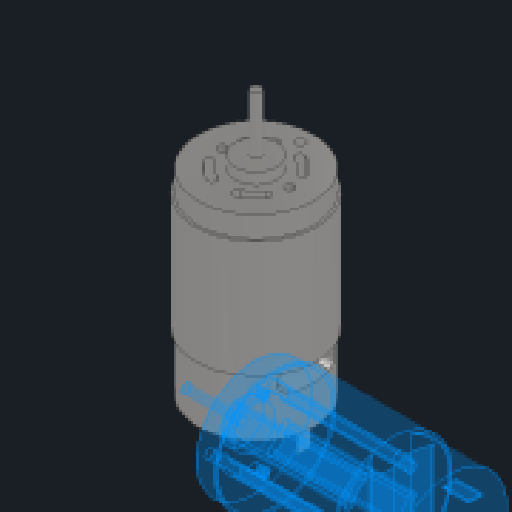
# Autodesk Inventor part: rs390
Saved by Autodesk Inventor 2023 (Build 270158000, 158)
## iProperties
Created: 2024-04-13
Part Number: rs390
Material: Steel, Mild
Document SubType Name: Modeling
Designer: szymo
Density: 3.82207 g/cm^3
Appearance: Semi-Polished
Mass: 100 g
Surface Area: 88.1627 cm^2
Volume: 26.1638 cm^3
Author: szymo
Autodesk Inventor part; units mm, degrees
ref_plane "YZ Plane" through (0, 0, 0) normal (1, 0, 0) x (0, 1, 0)
sketch "Sketch1" plane through (0, 0, 0) normal (0, 1, 0) x (-1, 0, 0)
  circle A0 centre (0, 0) radius 13.7
  dimension "d0" = 27.4
  constraints: 1 centre point, 1 coincident
  measures "d0" diameter of A0
extrude "Extrusion1" add sketch "Sketch1" along normal blind 46.5
sketch "Sketch2" plane through (0, 46.5, 0) normal (0, 1, 0) x (1, 0, 0)
  circle A0 centre (0, 0) radius 13.7 projected
  circle A1 centre (0, 0) radius 5
  dimension "d3" = 10
  constraints: 1 centre point, 1 coincident
  measures "d3" diameter of A1
extrude "Extrusion2" add sketch "Sketch2" along normal blind 2.7 contours A1
sketch "Sketch3" plane through (0, 46.5, 0) normal (0, 1, 0) x (1, 0, 0)
  circle A0 centre (0, 0) radius 5 projected
  circle A1 centre (0, 0) radius 5 projected
  circle A2 centre (0, 0) radius 13.7 projected
  circle A3 centre (0, 0) radius 13.7 projected
  line L0 (-13.7, 0) -> (13.7, 0)
  point P0 (-8, 0)
  point P1 (8, 0)
  dimension "d6" = 16
  dimension "d7" = 5.7
  dimension "d8" = 5.7
  constraints: 2 end point, 2 point on circle, 2 point on line, 1 horizontal
  measures "d6" distance of point (-8, 0) point (8, 0)
  measures "d7" distance of L0.start point (-8, 0)
  measures "d8" distance of L0.end point (8, 0)
hole "Hole1" at (-8, 46.5, 0) at (8, 46.5, 0) direction (0, -1, 0) diameter 2.1129 depth 2.8 thread size "M2.6x0.45" class "6H" standard "ISO Metric profile"
ref_plane "Work Plane1" through (0, 41.5, 0) normal (0, 1, 0) x (1, 0, 0)
sketch "Sketch4" plane through (0, 41.5, 0) normal (0, 1, 0) x (1, 0, 0)
  circle A0 centre (0, 0) radius 14.375
  dimension "d17" = 28.75
  constraints: 1 centre point, 1 coincident
  measures "d17" diameter of A0
extrude "Extrusion3" add sketch "Sketch4" against normal blind 27.7
sketch "Sketch5" plane through (0, 0, 0) normal (0, -1, 0) x (1, 0, 0)
  circle A0 centre (0, 0) radius 5
  dimension "d20" = 10
  constraints: 1 centre point, 1 coincident
  measures "d20" diameter of A0
extrude "Extrusion4" add sketch "Sketch5" along normal blind 4
sketch "Sketch6" plane through (0, 0, 0) normal (0, -1, 0) x (1, 0, 0)
  circle A0 centre (0, 0) radius 5 projected
  circle A1 centre (0, 0) radius 5 projected
  circle A2 centre (0, 0) radius 13.7 projected
  circle A3 centre (0, 0) radius 13.7 projected
  line L0 (13.7, 0) -> (-13.7, 0)
  line L1 (-11.5, 1.5) -> (-12, 1.5)
  line L2 (-12, 1.5) -> (-12, -1.5)
  line L3 (-12, -1.5) -> (-11.5, -1.5)
  line L4 (-11.5, -1.5) -> (-11.5, 1.5)
  line L5 (11.5, 1.5) -> (11, 1.5)
  line L6 (11, 1.5) -> (11, -1.5)
  line L7 (11, -1.5) -> (11.5, -1.5)
  line L8 (11.5, -1.5) -> (11.5, 1.5)
  dimension "d23" = 22.5
  dimension "d24" = 0.5
  dimension "d25" = 0.5
  dimension "d26" = 11.5
  dimension "d27" = 11.5
  dimension "d28" = 3
  dimension "d29" = 3
  dimension "d30" = 1.5
  dimension "d31" = 1.5
  constraints: 18 end point, 4 horizontal, 4 parallel, 2 perpendicular, 2 point on circle, 2 point on line
  measures "d23" distance between parallel lines of L6 L4
  measures "d24" distance of L6.end L7.end
  measures "d25" distance between parallel lines of L4 L2
  measures "d26" distance from line of A2.centre L8
  measures "d27" distance from line of A0.centre L4
  measures "d28" distance between parallel lines of L3 L1
  measures "d29" distance of L7.end L5.start
  measures "d30" distance between parallel lines of L0 L7
  measures "d31" distance between parallel lines of L0 L5
extrude "Extrusion5" add sketch "Sketch6" along normal blind 6 contours L6 L5 L8 L0 | L0 L8 L7 L6 | L4 L3 L2 L0 | L0 L2 L1 L4
sketch "Sketch7" plane through (0, 49.2, 0) normal (0, 1, 0) x (1, 0, 0)
  circle A0 centre (0, 0) radius 1.1
  dimension "d34" = 2.2
  constraints: 1 centre point, 1 coincident
  measures "d34" diameter of A0
extrude "Extrusion6" add sketch "Sketch7" along normal blind 13.5
ref_plane "Work Plane2" through (0, 50.2, 0) normal (0, 1, 0) x (1, 0, 0)
sketch "Sketch10" plane through (0, 0, 0) normal (1, 0, 0) x (0, 1, 0)
  line L0 (0, -13.7) -> (0, 13.7) projected
  line L1 (13.8, 13.7) -> (13.8, -13.7) projected
  line L2 (9, 4.6) -> (13.8, 4.6)
  line L3 (13.8, 4.6) -> (13.8, -4.6)
  line L4 (13.8, -4.6) -> (9, -4.6)
  line L5 (9, -4.6) -> (9, 4.6)
  circle A0 centre (11.4, 4.6) radius 2.4
  circle A1 centre (11.4, -4.6) radius 2.4
  line L6 (0, 0) -> (13.8, 0)
  line L7 (13.8, 13.7) -> (13.8, -13.7) projected
  line L8 (0, -13.7) -> (13.8, -13.7) projected
  point P0 (11.4, 7)
  point P1 (11.4, -7)
  point P2 (13.8, -4.6)
  dimension "d57" = 9
  dimension "d59" = 0
  dimension "d60" = 4.8
  dimension "d61" = 13.8
  dimension "d62" = 2.4
  dimension "d63" = 2.4
  dimension "d64" = 14
  dimension "d65" = 4.6
  dimension "d66" = 4.6
  dimension "d69" = 6.7
  constraints: 10 end point, 4 point on circle, 3 midpoint, 2 centre point, 2 parallel, 1 horizontal, 1 perpendicular
  measures "d57" distance between parallel lines of L0 L5
  measures "d59" distance between parallel lines of L3 L1
  measures "d60" distance between parallel lines of L5 L1
  measures "d61" distance between parallel lines of L0 L1
  measures "d62" distance from line of L4 A1.end
  measures "d63" distance from line of A0.end L2
  measures "d64" distance of A1.end A0.end
  measures "d65" distance from line of L6 A0.centre
  measures "d66" distance from line of L6 A1.centre
  measures "d69" distance from line of A1.end L8
extrude "Extrusion9" cut sketch "Sketch10" along normal mid plane 31.5 contours L6 L1 A1 L5 | L5 A0 L1 L6 | A1 L4 | L4 A1 | A0 L2 | L2 A0
sketch "Sketch11" plane through (0, 46.5, 0) normal (0, 1, 0) x (1, 0, 0)
  circle A0 centre (-8, 0) radius 1.0564 projected
  circle A1 centre (8, 0) radius 1.0564 projected
  circle A2 centre (0, 0) radius 5 projected
  circle A3 centre (0, 0) radius 13.7 projected
  circle A4 centre (8, 0) radius 1.0564 projected
  circle A5 centre (0, 0) radius 13.7 projected
  line L0 (13.7, 0) -> (-13.7, 0)
  circle A6 centre (0, 0) radius 1.1 projected
  circle A7 centre (0, 0) radius 9.0564
  circle A8 centre (0, 0) radius 6.9436
  circle A9 centre (8, 0) radius 1.0564 projected
  line L1 (1.8876, -9.0564) -> (-1.9124, -9.0564)
  line L2 (-1.9124, -9.0564) -> (-1.9124, 9.0564)
  line L3 (-1.9124, 9.0564) -> (1.8876, 9.0564)
  line L4 (1.8876, 9.0564) -> (1.8876, -9.0564)
  line L5 (-0.0124, -13.7) -> (-0.0124, 13.7)
  line L6 (9.0564, -3.15) -> (-9.0564, -3.15)
  line L7 (-9.0564, -3.15) -> (-9.0564, 3.15)
  line L8 (-9.0564, 3.15) -> (9.0564, 3.15)
  line L9 (9.0564, 3.15) -> (9.0564, -3.15)
  circle A10 centre (6.8048, -4.2064) radius 1.0564
  circle A11 centre (2.9441, -7.4386) radius 1.0564
  circle A12 centre (-2.9688, -7.4287) radius 1.0564
  circle A13 centre (-6.8048, -4.2064) radius 1.0564
  circle A14 centre (-6.8048, 4.2064) radius 1.0564
  line L10 (-11.7767, 7) -> (11.7767, 7) projected
  circle A15 centre (-2.9688, 7.4287) radius 1.0564
  circle A16 centre (2.9441, 7.4386) radius 1.0564
  circle A17 centre (6.8048, 4.2064) radius 1.0564
  circle A18 centre (-0.0124, 10.65) radius 1.15
  point P0 (9.0564, 0)
  point P1 (7.8048, -3.2064)
  point P2 (3.3328, 8.4209)
  point P3 (2.5553, 6.4563)
  point P4 (5.9062, 3.651)
  point P5 (7.7035, 4.7619)
  point P6 (-5.9062, 3.651)
  point P7 (-2.5768, 6.4477)
  point P8 (-3.3608, 8.4097)
  point P9 (-7.7035, 4.7619)
  point P10 (-3.3608, -8.4097)
  point P11 (-2.5768, -6.4477)
  point P12 (-5.9062, -3.651)
  point P13 (-7.7035, -4.7619)
  point P14 (7.7035, -4.7619)
  point P15 (5.9062, -3.651)
  point P16 (2.5553, -6.4563)
  point P17 (3.3328, -8.4209)
  point P18 (-0.0124, 11.8)
  dimension "d78" = 2.3
  dimension "d70" = 3.8
  dimension "d71" = 1.9
  dimension "d72" = 1.9
  dimension "d73" = 6.3
  dimension "d74" = 3.15
  dimension "d75" = 3.15
  dimension "d79" = 1.9
  constraints: 20 end point, 16 tangent, 9 centre point, 6 horizontal, 4 parallel, 4 point on circle, 3 perpendicular, 3 point on line, 3 vertical, 2 coincident, 2 horizontal alignment, 1 vertical alignment, 15 other
  measures "d70" distance of L2.end L3.end
  measures "d71" distance between parallel lines of L4 L5
  measures "d72" distance between parallel lines of L5 L2
  measures "d73" distance of L6.end L7.end
  measures "d74" distance between parallel lines of L6 L0
  measures "d75" distance between parallel lines of L0 L8
  measures "d79" distance of point (-0.012, 11.8) L5.end
extrude "Extrusion10" cut sketch "Sketch11" against normal blind 30 contours A14 A7 L10 A15 A8 | A14 | A8 A12 A7 A13 | A13 | A15 L10 | A12 | A7 A15 L10 | A15 L10 | A18 L5 | L5 A18 | L10 A16 A7 | A7 A17 A8 A16 L10 | A11 A8 A10 A7 | A11 | A17 | A16 L10 | A16 L10 | A10
equation "\"d7\" = d8"
equation "\"d26\" = d27"
equation "\"d30\" = d31"
equation "\"d65\" = d66"
equation "\"d71\" = d72"
equation "\"d74\" = d75"
equation "\"d41\" = d42"
body "Solid1"
